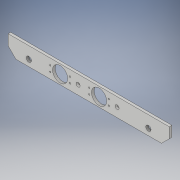
# Autodesk Inventor part: Drive Train - Smallest Model
Saved by Autodesk Inventor 2017 (Build 210142000, 142)
## iProperties
Created: 2017-08-02
Part Number: Drive Train - Smallest Model
Material: Generic
Document SubType Name: Modeling
Designer: User
Density: 1 g/cm^3
Appearance: Default
Author: User
Autodesk Inventor part; units mm, degrees
ref_plane "YZ Plane" through (0, 0, 0) normal (1, 0, 0) x (0, 1, 0)
ref_plane "XZ Plane" through (0, 0, 0) normal (0, 1, 0) x (-1, 0, 0)
ref_plane "XY Plane" through (0, 0, 0) normal (0, 0, 1) x (1, 0, 0)
sketch "Sketch1" plane through (0, 0, 0) normal (0, 0, 1) x (1, 0, 0)
  circle A0 centre (127, 19.05) radius 18.542
  circle A1 centre (222.25, 19.05) radius 18.542
  circle A2 centre (170.942, 19.05) radius 1.778
  circle A3 centre (266.192, 19.05) radius 1.778
  line L0 (151.003, 19.05) -> (151.003, 26.0604)
  circle A4 centre (102.997, 12.0396) radius 1.7526
  circle A5 centre (102.997, 26.0604) radius 1.7526
  circle A6 centre (151.003, 26.0604) radius 1.7526
  circle A7 centre (151.003, 12.0396) radius 1.7526
  line L1 (151.003, 19.05) -> (127, 19.05)
  circle A8 centre (246.253, 26.0604) radius 1.7526
  circle A9 centre (246.253, 12.0396) radius 1.7526
  circle A10 centre (198.247, 12.0396) radius 1.7526
  circle A11 centre (198.247, 26.0604) radius 1.7526
  line L2 (0, -3.175) -> (393.7, -3.175)
  line L3 (0, 41.275) -> (393.7, 41.275)
  line L4 (0, 41.275) -> (0, -3.175)
  line L5 (393.7, 41.275) -> (393.7, -3.175)
  circle A12 centre (222.25, 19.05) radius 18.542
  circle A13 centre (246.253, 26.0604) radius 1.7526
  circle A14 centre (246.253, 12.0396) radius 1.7526
  circle A15 centre (266.192, 19.05) radius 1.778
  circle A16 centre (198.247, 12.0396) radius 1.7526
  circle A17 centre (198.247, 26.0604) radius 1.7526
  circle A18 centre (170.942, 19.05) radius 1.778
  circle A19 centre (151.003, 12.0396) radius 1.7526
  circle A20 centre (151.003, 26.0604) radius 1.7526
  circle A21 centre (127, 19.05) radius 18.542
  circle A22 centre (102.997, 12.0396) radius 1.7526
  circle A23 centre (102.997, 26.0604) radius 1.7526
  circle A24 centre (50.8, 12.7) radius 6.35
  circle A25 centre (342.9, 12.7) radius 6.35
  point P0 (0, 0)
  dimension "d3" = 37.084
  dimension "d5" = 37.084
  dimension "d10" = 3.556
  dimension "d11" = 3.556
  dimension "d24" = 7.0104
  dimension "d28" = 3.5052
  dimension "d29" = 3.5052
  dimension "d30" = 3.5052
  dimension "d31" = 24.003
  dimension "d38" = 3.5052
  dimension "d39" = 3.5052
  dimension "d40" = 3.5052
  dimension "d41" = 3.5052
  constraints: 26 centre point, 15 coincident, 12 concentric, 12 end point, 3 horizontal, 3 vertical
  measures "d3" diameter of A0
  measures "d5" diameter of A1
  measures "d10" diameter of A2
  measures "d11" diameter of A3
  measures "d24" distance of L0.start L0.end
  measures "d28" diameter of A4
  measures "d29" diameter of A5
  measures "d30" diameter of A6
  measures "d31" distance of L0.start L1.end
  measures "d38" diameter of A8
  measures "d39" diameter of A9
  measures "d40" diameter of A10
  measures "d41" diameter of A11
extrude "Extrusion4" add sketch "Sketch1" along normal blind 6.35 contours L4 L3 L5 L2 | A24 | A25
chamfer "Chamfer2" distance 3.175 angle 45 2 edges at (169.164, 19.05, 6.35) (264.414, 19.05, 6.35)
extrude "Extrusion5" cut sketch "Sketch1" along normal blind 25.4 contours A24 | A25
chamfer "Chamfer3" distance 19.05 angle 45 1 edges at (0, -3.175, 3.175)
chamfer "Chamfer4" distance 19.05 angle 45 1 edges at (393.7, -3.175, 3.175)
body "Solid1"
